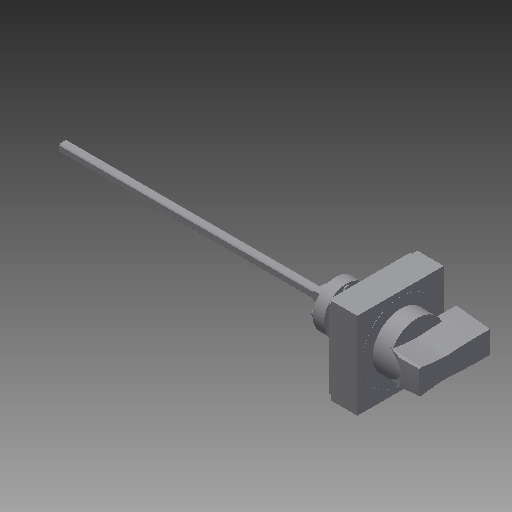
# Autodesk Inventor part: 100031(5,310)_P1
Saved by Autodesk Inventor 2019.3 (Build 233278000, 278)
## iProperties
Category: PARTsolutions
Company: MOELLER
Created: 2018-12-14
Part Number: 100031(5,310)_P1
Material: Generic
Catalog Web Link: www.cadenas.de
Description: NZM1-XS Part1-NZM1-XS
Vendor: MOELLER
Document SubType Name: Modeling
Designer: psadmin
Manufacturer: MOELLER
Mass: 332.142 g
Surface Area: 486.841 cm^2
Volume: 332.142 cm^3
Density: 1 g/cm^3
Appearance: PSOLRGB-192-192-192
PSOL_IDENT_0: {$CADENAS_DATA\23d-libs\moeller\circuit_breaker\parts\nzm1_xs_p1.prj},187 {VTYP=3D},{NB=100031(5,310
PSOL_IDENT_1: )_P1},{LINA=100031(5,310)_P1},{NN=NZM1-XS Part1},{DATE=10.12.2018 21:08:04},{GEOMDATE=14.05.2018 10:
PSOL_IDENT_2: 43:05},{VERSION=},{LINEID=60},{WBVAR=BS,L},{WBNUMERIC=BS,L}  {NB=100031(5,310)_P1},{LINA=100031(5,31
PSOL_IDENT_3: 0)_P1},{KT=DUMMY},{BMENB=100031},{BS=5},{L=310},{VER=2},{EPLAN=}
NN: NZM1-XS Part1
NT: NZM1-XS
NB: 100031(5,310)_P1
NBSYN: $BMENB.($BS.,$L.)_P1
LINA: 100031(5,310)_P1
BMENB: 100031
BS: 5
L: 310
VER: 2
SUPPLIER: MOELLER
ARTICLENO: 100031(5,310)_P1
BOMINFO: 100031(5,310)_P1
CREATOR: CADENAS GmbH
Title: 100031(5,310)_P1
Author: Cadenas PARTsolutions
Comments: NZM1-XS
Autodesk Inventor part; units mm, degrees
sketch "Sketch_6" plane through (35.8, 0, 0) normal (1, 0, 0) x (0, 0, -1)
  arc A0 (-28.0821, 12.97) -> (-28.0821, -12.97) centre (173, 0) ccw
  line L0 (-28.0821, -12.97) -> (-24.14, -13.9317)
  arc A1 (0.1108, -11.3777) -> (-24.14, -13.9317) centre (5.9, -182.76) ccw
  arc A2 (0.1108, -11.3777) -> (44.85, -12.6864) centre (36.04, 451.53) ccw
  line L1 (44.85, -12.6864) -> (44.85, 12.6864)
  arc A3 (44.85, 12.6864) -> (0.1108, 11.3777) centre (36.04, -451.53) ccw
  arc A4 (-24.14, 13.9317) -> (0.1108, 11.3777) centre (5.9, 182.76) ccw
  line L2 (-24.14, 13.9317) -> (-28.0821, 12.97)
  constraints: 10 point on circle, 6 end point, 5 centre point
extrude "Extrusion1" add sketch "Sketch_6" along normal blind 35 draft -3
sketch "Sketch_9" plane through (0, 0, 0) normal (0, 1, 0) x (-1, 0, 0)
  line L0 (-35.8, 22.92) -> (-35.8, 29.9)
  line L1 (-35.8, 29.9) -> (-54.8, 27.9)
  line L2 (-54.8, 27.9) -> (-35.8, 22.92)
  constraints: 6 end point
extrude "Extrusion2" cut sketch "Sketch_9" along normal mid plane 40
sketch "Sketch_8" plane through (0, 0, 0) normal (0, 0, 1) x (1, 0, 0)
  line L0 (42.15, 0) -> (25.9, 0)
  line L1 (25.9, 0) -> (25.9, 27.5)
  line L2 (25.9, 27.5) -> (42.15, 27.5)
  line L3 (42.15, 27.5) -> (42.15, 0)
  line L4 (42.15, 0) -> (25.9, 0)
  constraints: 10 end point
revolve "Revolution1" add sketch "Sketch_8" angle 360 about axis through (42.15, 0, 0) along (1, 0, 0)
sketch "Sketch_10" plane through (0, 0, 0) normal (0, 1, 0) x (-1, 0, 0)
  line L0 (-25.9, 0) -> (-53.65, 0)
  line L1 (-53.65, 0) -> (-53.65, 27.5)
  line L2 (-53.65, 27.5) -> (-25.9, 27.5)
  line L3 (-25.9, 27.5) -> (-25.9, 0)
  line L4 (-25.9, 0) -> (-53.65, 0)
  constraints: 10 end point
revolve "Revolution2" add sketch "Sketch_10" angle 56 mid plane about axis through (25.9, 0, 0) along (1, 0, 0)
sketch "Sketch_3" plane through (0, 0, 0) normal (1, 0, 0) x (0, 1, 0)
  line L0 (-42.5, 42.5) -> (-42.5, -42.5)
  line L1 (-42.5, -42.5) -> (42.5, -42.5)
  line L2 (42.5, -42.5) -> (42.5, 42.5)
  line L3 (42.5, 42.5) -> (-42.5, 42.5)
  constraints: 8 end point
extrude "Extrusion3" add sketch "Sketch_3" along normal blind 25.9
sketch "Sketch_4" plane through (0, 0, 0) normal (0, 0, 1) x (1, 0, 0)
  line L0 (23.9, 0) -> (25.9, 0)
  line L1 (23.9, -37.7) -> (25.9, -37.7)
  line L2 (25.9, -37.7) -> (25.9, -37.5)
  line L3 (25.9, -37.5) -> (23.9, -37.5)
  line L4 (23.9, -37.5) -> (23.9, -37.7)
  constraints: 10 end point
revolve "Revolution3" cut sketch "Sketch_4" angle 360 about axis through (23.9, 0, 0) along (-1, 0, 0)
sketch "Sketch_2" plane through (0, 0, 0) normal (1, 0, 0) x (0, 1, 0)
  line L0 (-38.5, 41.5) -> (-41.5, 38.5)
  line L1 (-41.5, 38.5) -> (-41.5, -38.5)
  line L2 (-41.5, -38.5) -> (-38.5, -41.5)
  line L3 (-38.5, -41.5) -> (38.5, -41.5)
  line L4 (38.5, -41.5) -> (41.5, -38.5)
  line L5 (41.5, -38.5) -> (41.5, 38.5)
  line L6 (41.5, 38.5) -> (38.5, 41.5)
  line L7 (38.5, 41.5) -> (-38.5, 41.5)
  constraints: 16 end point
extrude "Extrusion4" add sketch "Sketch_2" against normal blind 3
sketch "Sketch_1" plane through (0, 0, 0) normal (0, 0, 1) x (1, 0, 0)
  line L0 (0, 0) -> (-46, 0)
  line L1 (-46, 0) -> (-46, 4.5)
  line L2 (-46, 4.5) -> (-38, 4.5)
  line L3 (-38, 4.5) -> (-38, 22.5)
  line L4 (-38, 22.5) -> (-27, 22.5)
  line L5 (-27, 22.5) -> (-27, 4.5)
  line L6 (-27, 4.5) -> (0, 4.5)
  line L7 (0, 4.5) -> (0, 0)
  line L8 (0, 0) -> (-46, 0)
  constraints: 18 end point
revolve "Revolution4" add sketch "Sketch_1" angle 360 about axis through (0, 0, 0) along (1, 0, 0)
sketch "Sketch_7" plane through (0, 0, 0) normal (0, 1, 0) x (-1, 0, 0)
  line L0 (38, -17) -> (40.8, -17)
  line L1 (40.8, -17) -> (40.8, -21)
  line L2 (40.8, -21) -> (38, -21)
  line L3 (38, -21) -> (38, -17)
  line L4 (38, -17) -> (40.8, -17)
  constraints: 10 end point
revolve "Revolution5" add sketch "Sketch_7" angle 360 about axis through (-38, 0, -17) along (1, 0, 0)
sketch "Sketch_11" plane through (0, 0, 0) normal (0, 1, 0) x (-1, 0, 0)
  line L0 (38, 17) -> (40.8, 17)
  line L1 (40.8, 17) -> (40.8, 13)
  line L2 (40.8, 13) -> (38, 13)
  line L3 (38, 13) -> (38, 17)
  line L4 (38, 17) -> (40.8, 17)
  constraints: 10 end point
revolve "Revolution6" add sketch "Sketch_11" angle 360 about axis through (-38, 0, 17) along (1, 0, 0)
sketch "Sketch_12" plane through (0, 0, 0) normal (0, 0, 1) x (1, 0, 0)
  line L0 (-25.8, 17) -> (-27, 17)
  line L1 (-27, 17) -> (-27, 21)
  line L2 (-27, 21) -> (-25.8, 21)
  line L3 (-25.8, 21) -> (-25.8, 17)
  line L4 (-25.8, 17) -> (-27, 17)
  constraints: 10 end point
revolve "Revolution7" add sketch "Sketch_12" angle 360 about axis through (-25.8, 17, 0) along (1, 0, 0)
sketch "Sketch_13" plane through (0, 0, 0) normal (0, 0, 1) x (1, 0, 0)
  line L0 (-25.8, -17) -> (-27, -17)
  line L1 (-27, -17) -> (-27, -13)
  line L2 (-27, -13) -> (-25.8, -13)
  line L3 (-25.8, -13) -> (-25.8, -17)
  line L4 (-25.8, -17) -> (-27, -17)
  constraints: 10 end point
revolve "Revolution8" add sketch "Sketch_13" angle 360 about axis through (-25.8, -17, 0) along (1, 0, 0)
sketch "Sketch_14" plane through (-38, 0, 0) normal (1, 0, 0) x (0, 0, -1)
  line L0 (-6.1, -2.668) -> (-2.668, -6.1)
  line L1 (-2.668, -6.1) -> (6.1, -6.1)
  line L2 (6.1, -6.1) -> (6.1, 6.1)
  line L3 (6.1, 6.1) -> (-6.1, 6.1)
  line L4 (-6.1, 6.1) -> (-6.1, -2.668)
  line L5 (-4.6, -2.047) -> (-2.047, -4.6)
  line L6 (-2.047, -4.6) -> (4.6, -4.6)
  line L7 (4.6, -4.6) -> (4.6, 4.6)
  line L8 (4.6, 4.6) -> (-4.6, 4.6)
  line L9 (-4.6, 4.6) -> (-4.6, -2.047)
  constraints: 20 end point
extrude "Extrusion5" add sketch "Sketch_14" along normal mid plane 32
sketch "Sketch_15" plane through (-38, 0, 0) normal (1, 0, 0) x (0, 0, -1)
  line L0 (-6.1, -2.668) -> (-2.668, -6.1)
  line L1 (-2.668, -6.1) -> (6.1, -6.1)
  line L2 (6.1, -6.1) -> (6.1, 6.1)
  line L3 (6.1, 6.1) -> (-6.1, 6.1)
  line L4 (-6.1, 6.1) -> (-6.1, -2.668)
  constraints: 10 end point
extrude "Extrusion6" add sketch "Sketch_15" along normal mid plane 16
sketch "Sketch_16" plane through (-46, 0, 0) normal (1, 0, 0) x (0, 0, -1)
  arc A0 (-4, -2.5617) -> (-2.5617, -4) centre (0, 0) ccw
  line L0 (-2.5617, -4) -> (2.5617, -4)
  arc A1 (2.5617, -4) -> (4, -2.5617) centre (0, 0) ccw
  line L1 (4, -2.5617) -> (4, 2.5617)
  arc A2 (4, 2.5617) -> (2.5617, 4) centre (0, 0) ccw
  line L2 (2.5617, 4) -> (-2.5617, 4)
  arc A3 (-2.5617, 4) -> (-4, 2.5617) centre (0, 0) ccw
  line L3 (-4, 2.5617) -> (-4, -2.5617)
  constraints: 8 end point, 8 point on circle, 4 centre point
extrude "Extrusion7" add sketch "Sketch_16" against normal blind 259.5
ref_plane "P1_XY" through (-3, 0, 0) normal (1, 0, 0) x (0, 0, -1)
ref_plane "P1_YZ" through (-3, 0, 0) normal (0, 0, -1) x (0, 1, 0)
ref_plane "P1_ZX" through (-3, 0, 0) normal (0, 1, 0) x (1, 0, 0)
ref_plane "P1_to_P3_XY" through (-305.5, 0, 0) normal (1, 0, 0) x (0, 0, -1)
ref_plane "P1_to_P3_YZ" through (-305.5, 0, 0) normal (0, 0, -1) x (0, 1, 0)
ref_plane "P1_to_P3_ZX" through (-305.5, 0, 0) normal (0, 1, 0) x (1, 0, 0)
body "Solid1"
